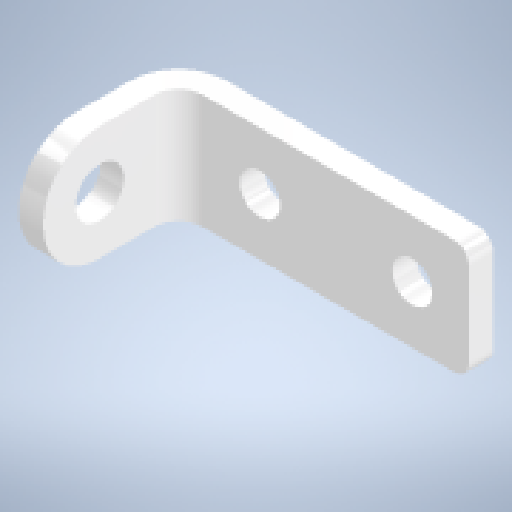
# Autodesk Inventor part: Inductive Sensor Bracket
Saved by Autodesk Inventor 2024 (Build 280153000, 153)
## iProperties
Created: 2025-01-01
Part Number: Inductive Sensor Bracket
Material: Aluminum 6061
Document SubType Name: Sheet Metal
Designer: Ishaan
Density: 2.7 g/cm^3
Sheet Metal Rule: SendCutSend_1-8_Alu
Appearance: Aluminum - Flat
Author: Ishaan
Autodesk Inventor part; units mm, degrees
ref_plane "YZ Plane" through (0, 0, 0) normal (1, 0, 0) x (0, 1, 0)
ref_plane "XZ Plane" through (0, 0, 0) normal (0, 1, 0) x (-1, 0, 0)
ref_plane "XY Plane" through (0, 0, 0) normal (0, 0, 1) x (1, 0, 0)
sketch "Sketch1" plane through (0, 0, 0) normal (0, 0, 1) x (1, 0, 0)
  line L0 (17.5, -7.5) -> (-17.5, -7.5)
  line L1 (-17.5, -7.5) -> (-17.5, 7.5)
  line L2 (-17.5, 7.5) -> (17.5, 7.5)
  line L3 (17.5, 7.5) -> (17.5, -7.5)
  line L4 (17.5, -7.5) -> (-17.5, 7.5) construction
  line L5 (-17.5, -7.5) -> (17.5, 7.5) construction
  line L6 (-10, 0) -> (10, 0) construction
  point P0 (0, 0)
  dimension "d0" = 35
  dimension "d1" = 15
  dimension "d2" = 20
  dimension "d3" = 7.5
  constraints: 14 end point, 3 midpoint, 2 horizontal, 2 parallel, 1 perpendicular
  measures "d0" distance of L1.end L2.end
  measures "d1" distance of L0.end L1.end
  measures "d2" distance of L6.start L6.end
  measures "d3" distance from line of L6.end L3
extrude "Plate1" add sketch "Sketch1" along normal blind 3.175
sketch "Sketch2" plane through (-20.675, -7.5, 6.35) normal (-1, 0, 0) x (0, -1, 0)
  line L0 (-15, 0) -> (0, 0)
  line L1 (0, 0) -> (0, 13.65)
  line L2 (0, 13.65) -> (-15, 13.65)
  line L3 (-15, 13.65) -> (-15, 0)
  constraints: 6 end point, 1 horizontal, 1 perpendicular, 1 vertical
edge flange "Flange1" height 20 angle 90 thickness 3.175 bend radius 3.175 thickness toward (-1, 0, 0) relief tear relief width 3.175 relief depth 1.5875 edges at (-17.5, 0, 3.175) wall of the first edge with corners at (-20.675, 7.5, 6.35) (-20.675, -7.5, 6.35) (-20.675, -7.5, 20) (-20.675, 7.5, 20)
bend "Bend1"
corner "Corner1"
hole "Hole1" at (-10, 0, 0) at (10, 0, 0) direction (0, 0, 1) diameter 5.3 end through all
sketch "Sketch3" plane through (-20.675, -7.5, 20) normal (1, 0, 0) x (0, 0, -1)
  line L0 (13.65, 0) -> (13.65, 15) projected
  line L1 (0, 15) -> (13.65, 15) projected
  line L2 (0, 15) -> (0, 0) projected
  line L3 (0, 0) -> (13.65, 0) projected
  circle A0 centre (7.5, 7.5) radius 7.5
  point P0 (20, 7.5)
  point P1 (0, 7.5)
  point P2 (7.5, 15)
  point P3 (7.5, 0)
  constraints: 3 tangent, 1 centre point
hole "Hole2" at (-20.675, 0, 12.5) direction (-1, 0, 0) diameter 6.4 end through all
extrude "Extrusion1" cut sketch "Sketch3" against normal through all contours L3 L2 A0 | L2 L1 A0
fillet "Fillet1" radius 2 2 edges at (17.5, 7.5, 1.5875) (17.5, -7.5, 1.5875)
equation "\"d0\" = d2 + d1"
equation "\"d3\" = 0.5 * d1"
equation "\"d20\" = Thickness"
equation "\"d4\" = Thickness"
equation "\"d5\" = BendReliefWidth"
equation "\"d6\" = BendReliefDepth"
equation "\"d7\" = MinimumRemnant"
equation "\"d8\" = TransitionRadius"
equation "\"d11\" = BendRadius"
equation "\"d12\" = CornerReliefSize"
equation "\"d13\" = GapSize"
equation "\"d14\" = JacobiRadiusSize"
equation "\"BendReliefWidth\" = Thickness"
equation "\"BendReliefDepth\" = 0.5 * Thickness"
equation "\"CornerReliefSize\" = 4 * Thickness"
equation "\"MinimumRemnant\" = 2 * Thickness"
equation "\"TransitionRadius\" = BendRadius"
equation "\"JacobiRadiusSize\" = BendRadius"
equation "\"GapSize\" = Thickness"
equation "\"Thickness\" = 3.175"
equation "\"BendRadius\" = 3.175"
body "Solid1"
